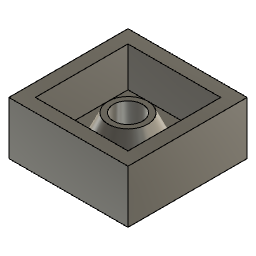
PenHolder (Autodesk Fusion 360 design; units mm, degrees)
Autodesk Fusion 360 part; units mm, degrees
sketch "Sketch1" plane through (0, 0, 0) normal (0, 0, 1) x (1, 0, 0)
  line L0 (-22.5, 22.5) -> (22.5, 22.5)
  line L1 (22.5, 22.5) -> (22.5, -22.5)
  line L2 (22.5, -22.5) -> (-22.5, -22.5)
  line L3 (-22.5, -22.5) -> (-22.5, 22.5)
  line L4 (-22.5, 22.5) -> (22.5, -22.5) construction
  dimension "d1" = 45
  constraint horizontal L0
  constraint vertical L1
  constraint horizontal L2
  constraint vertical L3
  constraint midpoint origin L4
  constraint equal L0 L3
  measures "d1" horizontal distance of L0.start L1.end
extrude "Extrude1" add sketch "Sketch1" along normal blind 20
sketch "Sketch2" plane through (0, 0, 20) normal (0, 0, 1) x (-1, 0, 0)
  line L0 (22.5, 22.5) -> (-22.5, 22.5)
  line L1 (-22.5, 22.5) -> (-22.5, -22.5)
  line L2 (-22.5, -22.5) -> (22.5, -22.5)
  line L3 (22.5, -22.5) -> (22.5, 22.5)
  line L4 (-17.5, -17.5) -> (17.5, -17.5)
  line L5 (17.5, -17.5) -> (17.5, 17.5)
  line L6 (17.5, 17.5) -> (-17.5, 17.5)
  line L7 (-17.5, 17.5) -> (-17.5, -17.5)
  line L8 (-17.5, -17.5) -> (17.5, 17.5) construction
  line L9 (17.5, -17.5) -> (-17.5, 17.5) construction
  dimension "d4" = 5
  dimension "d5" = 5
  constraint horizontal L4
  constraint perpendicular L4 L5
  constraint parallel L4 L6
  constraint parallel L5 L7
  constraint coincident L8 origin
  constraint coincident L9 origin
  measures "d4" distance of L1 L7
  measures "d5" distance of L2 L4
extrude "Extrude2" cut sketch "Sketch2" against normal blind 15 contours L4 L5 L6 L7
sketch "Sketch3" plane through (0, 0, 0) normal (0, 1, 0) x (1, 0, 0)
  line L0 (22.5, -20) -> (22.5, 0)
  line L1 (22.5, 0) -> (-22.5, 0)
  line L2 (-22.5, 0) -> (-22.5, -20)
  line L3 (-22.5, -20) -> (-17.5, -20)
  line L4 (-17.5, -20) -> (-17.5, -5)
  line L5 (-17.5, -5) -> (17.5, -5)
  line L6 (17.5, -5) -> (17.5, -20)
  line L7 (17.5, -20) -> (22.5, -20)
  line L8 (-7.5, -15) -> (7.5, -15)
  line L9 (0, -15) -> (0, -5) construction
  line L10 (-7.5, -15) -> (-12.1631, -5)
  line L11 (7.5, -15) -> (12.1631, -5)
  line L12 (-5.5, -15) -> (5.5, -15)
  line L13 (5.5, -15) -> (5.5, -5)
  line L14 (5.5, -5) -> (-5.5, -5)
  line L15 (-5.5, -5) -> (-5.5, -15)
  dimension "d8" = 15
  dimension "d9" = 65
  dimension "d10" = 65
  dimension "d11" = 11
  dimension "d12" = 10
  constraint horizontal L8
  constraint midpoint L8 L9.start
  constraint midpoint L5 L9.end
  constraint vertical L9
  constraint coincident L5 L10.end
  constraint coincident L5 L11.end
  constraint horizontal L12
  constraint vertical L13
  constraint horizontal L14
  constraint vertical L15
  constraint coincident L5 L13.end
  constraint coincident L8 L12.start
  constraint midpoint L8 L12
  measures "d8" distance of L8.start L8.end
  measures "d9" angle of L5 L10
  measures "d10" angle of L5 L11
  measures "d11" distance of L13 L15
  measures "d12" distance of L5 L8
revolve "Revolve1" add sketch "Sketch3" angle 360 about axis through (0, 0, 15) along (0, 0, -1) contours L5 L8 L10 L15
